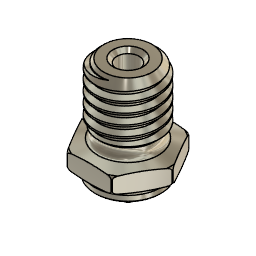
FIN 0.4mm Nozzle (Threads) (Autodesk Fusion 360 design; units mm, degrees)
Autodesk Fusion 360 part; units mm, degrees
note: some values were not read from the file. Set by a fixed rule: which sketch regions a step uses.
sketch "Revolve Sketch" plane through (0, 0, 0) normal (0, 1, 0) x (1, 0, 0)
  line L0 (-0.2, 0) -> (-0.4, 0)
  arc A0 (-0.4, 0) -> (-0.5226, -0.0572) centre (-0.4, -0.16) ccw
  line L1 (-0.5226, -0.0572) -> (-1.5834, -1.3214)
  arc A1 (-1.9664, -1.5) -> (-1.5834, -1.3214) centre (-1.9664, -1) ccw
  line L2 (-1.9664, -1.5) -> (-2.5, -1.5)
  arc A2 (-2.5, -1.5) -> (-2.6, -1.6) centre (-2.5, -1.6) ccw
  line L3 (-2.6, -1.6) -> (-2.6, -2)
  arc A3 (-2.9706, -2.483) -> (-2.6, -2) centre (-3.1, -2) ccw
  line L4 (-2.9706, -2.483) -> (-3.3518, -2.5851)
  arc A4 (-3.5, -3.6217) -> (-3.3518, -3.8149) centre (-3.3, -3.6217) ccw
  line L5 (-3.3518, -3.8149) -> (-2.3706, -4.0778)
  arc A5 (-3.3518, -2.5851) -> (-3.5, -2.7783) centre (-3.3, -2.7783) ccw
  line L6 (-3.5, -2.7783) -> (-3.5, -3.6217)
  line L7 (-0.2, 0) -> (-0.2, -1)
  line L8 (-0.2, -1) -> (-0.875, -1.8044)
  line L9 (-0.875, -1.8044) -> (-0.875, -9.5)
  line L10 (0, 0) -> (0, -9.5) construction
  arc A6 (-2.1464, -4.9143) -> (-2.3706, -4.0778) centre (-2.5, -4.5608) ccw
  line L11 (-2.1464, -4.9143) -> (-2.5, -5.2679)
  line L12 (-2.5, -5.2679) -> (-2.5, -8.9)
  line L13 (-2.5, -8.9) -> (-1.9, -9.5)
  line L14 (-1.9, -9.5) -> (-1.175, -9.5)
  line L15 (2.5, -11.5) -> (4.5, -11.5)
  line L16 (4.5, -11.5) -> (4.5, -4.5608)
  line L17 (4.5, -4.5608) -> (2.5, -4.5608)
  line L18 (2.5, -4.5608) -> (2.5, -11.5)
  line L19 (-1.175, -9.5) -> (-0.875, -9.2)
  point P0 (-5.6466, -3.2)
  dimension "d1" = 7
  dimension "d2" = 0.2
  dimension "d3" = 0.5
  dimension "d4" = 0.1
  dimension "d5" = 0.5
  dimension "d6" = 0.16
  dimension "d7" = 0.4
  dimension "d8" = 0.2
  dimension "d9" = 40
  dimension "d10" = 1.5
  dimension "d11" = 5.2
  dimension "d12" = 2
  dimension "d13" = 15
  dimension "d14" = 30
  dimension "d15" = 3.2
  dimension "d16" = 0.5
  dimension "d17" = 2
  dimension "d18" = 1.75
  dimension "d19" = 1
  dimension "d20" = 40
  dimension "d21" = 3.8
  dimension "d22" = 9.5
  dimension "d23" = 45
  dimension "d24" = 5
  dimension "d25" = 60
  dimension "d30" = 2
  dimension "d31" = 2
  dimension "d36" = 45
  dimension "d37" = 0.3
  constraint horizontal L0
  constraint tangent L0 A0
  constraint tangent A0 L1
  constraint tangent L1 A1
  constraint tangent L2 A2
  constraint tangent L3 A3
  constraint tangent L4 A5
  constraint tangent A4 L6
  constraint tangent A4 L5
  constraint tangent A5 L6
  constraint tangent A3 L4
  constraint tangent A2 L3
  constraint tangent A1 L2
  constraint perpendicular L0 L7
  constraint perpendicular L0 L9
  constraint coincident L10.start origin
  constraint vertical L10
  constraint vertical L6
  constraint equal A4 A5
  constraint horizontal L2
  constraint vertical L3
  constraint coincident L0 L10.start
  constraint coincident L5 P0
  constraint coincident L4 P0
  constraint tangent L5 A6
  constraint tangent A6 L11
  constraint coincident L10.end L14
  constraint vertical L12
  constraint horizontal L14
  constraint horizontal L15
  constraint vertical L16
  constraint horizontal L17
  constraint vertical L18
  constraint coincident A6.centre L17
  constraint coincident L9 L19.end
  measures "d2" radius of A5
  measures "d3" radius of A3
  measures "d4" radius of A2
  measures "d5" radius of A1
  measures "d6" radius of A0
  measures "d8" distance of L0.start L0.end
  measures "d9" angle of L1 L10
  measures "d10" distance of L0 L2
  measures "d12" distance of L0 A3.centre
  measures "d13" angle of L0 L4
  measures "d14" angle of L4 L5
  measures "d15" distance of L0 P0
  measures "d16" radius of A6
  measures "d17" distance of L10 A6
  measures "d19" distance of L0.start L7.end
  measures "d20" angle of L8 L10
  measures "d22" distance of L10.start L10.end
  measures "d23" angle of L13 L14
  measures "d25" angle of L5 L11
  measures "d30" distance of L10.end L15
  measures "d31" distance of L15.start L15.end
  measures "d36" angle of L14 L19
  measures "d37" horizontal distance of L14.end L19.end
revolve "Revolve1" add sketch "Revolve Sketch" angle 360 about axis through (0, 0, 0) along (0, 0, 1) contours L0 A0 L1 A1 L2 A2 L3 A3 L4 A4 L5 A5 L6 L7 L8 L9 A6 L11 L12 L13 L14 L19 makes body 1
sketch "Hex Cut" plane through (0, 0, 0) normal (0, 0, 1) x (1, 0, 0)
  circle A0 centre (0, 0) radius 5
  line L0 (1.7609, -3.05) -> (3.5218, 0)
  line L1 (3.5218, 0) -> (1.7609, 3.05)
  line L2 (1.7609, 3.05) -> (-1.7609, 3.05)
  line L3 (-1.7609, 3.05) -> (-3.5218, 0)
  line L4 (-3.5218, 0) -> (-1.7609, -3.05)
  line L5 (-1.7609, -3.05) -> (1.7609, -3.05)
  dimension "d27" = 10
  dimension "d28" = 6.1
  constraint coincident A0.centre origin
  constraint horizontal L5
  measures "d27" diameter of A0
  measures "d28" distance of L2 L5
extrude "Extrude1" cut sketch "Hex Cut" along normal through all bodies 1
revolve "Revolve2" add sketch "Revolve Sketch" angle 360 about axis through (0, 0, 0) along (0, 0, 1) separate body contours L15 L16 L17 L18 makes body 2
thread "Thread1" "ISO Metric profile 5.0 M5x0.8 6H" major diameter 5.12 minor diameter 4.234 pitch 0.8 angle 60 modelled right hand crest width 0.2219 on face at (2.4876, -0.2489, 6.8738) crest through (2.117, 0, 4.7608) on bodies 2
combine "Combine1" operation cut target body 1 tool bodies 2
equation "d6 = 0.4 * NozzleDiameter"
equation "d7 = NozzleDiameter"
equation "d8 = d7 * 0.5"
equation "d17 = ( 4 / 2 ) * 1 mm"
equation "NozzleDiameter = 0.4 mm"
named bodies: "FIN 0.4mm Nozzle"
